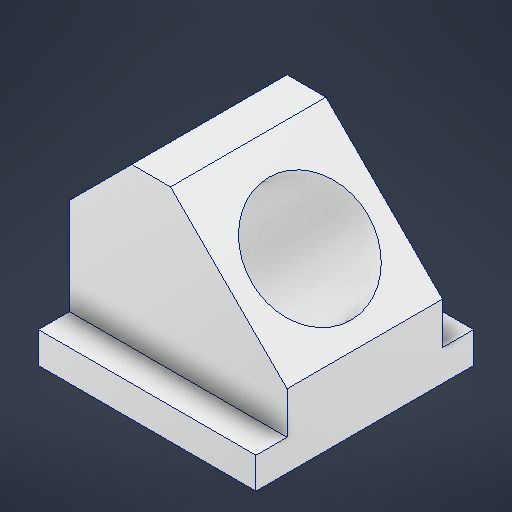
# Autodesk Inventor part: MMAE 232 - Assignment 1a-Nicholas Skiba
Saved by Autodesk Inventor 2026.1 (Build 301233000, 233)
## iProperties
Created: 2025-08-25
Part Number: MMAE 232 - Assignment 1a-Nicholas Skiba
Material: Aluminum 6061
Document SubType Name: Modeling
Designer: Nick
Density: 2.7 g/cm^3
Appearance: Aluminum - Flat
Mass: 20806.1 g
Surface Area: 3990.36 cm^2
Volume: 7705.95 cm^3
Author: Nick
Autodesk Inventor part; units mm, degrees
ref_plane "YZ Plane" through (0, 0, 0) normal (1, 0, 0) x (0, 1, 0)
ref_plane "XZ Plane" through (0, 0, 0) normal (0, 1, 0) x (-1, 0, 0)
ref_plane "XY Plane" through (0, 0, 0) normal (0, 0, 1) x (1, 0, 0)
sketch "Sketch1" plane through (0, 0, 0) normal (0, 1, 0) x (-1, 0, 0)
  line L0 (0, 0) -> (280, 0)
  line L1 (280, 0) -> (280, -280)
  line L2 (280, -280) -> (0, -280)
  line L3 (0, -280) -> (0, 0)
  line L4 (0, 0) -> (0, -20)
  line L5 (0, -20) -> (280, -20)
  line L6 (280, -20) -> (280, -260)
  line L7 (280, -260) -> (0, -260)
  line L8 (0, -260) -> (0, -20)
  dimension "d0" = 280
  dimension "d1" = 280
  dimension "d2" = 20
  dimension "d3" = 240
  constraints: 18 end point, 4 parallel, 2 horizontal, 2 perpendicular, 2 point on line
  measures "d0" distance of L1.end L2.end
  measures "d1" distance of L0.end L1.end
  measures "d2" distance of L0.start L4.end
  measures "d3" distance of L5.end L6.end
extrude "Extrusion1" add sketch "Sketch1" along normal blind 244 contours L5 L1 L7 L3
sketch "Sketch2" plane through (0, 0, 0) normal (0, -1, 0) x (1, 0, 0)
  line L0 (0, 0) -> (-280, 0)
  line L1 (-280, 0) -> (-280, -280)
  line L2 (-280, -280) -> (0, -280)
  line L3 (0, -280) -> (0, 0)
  dimension "d6" = 280
  dimension "d7" = 280
  constraints: 8 end point, 2 parallel, 1 horizontal, 1 perpendicular
  measures "d6" distance of L2.end L1.end
  measures "d7" distance of L1.end L0.end
extrude "Extrusion2" add sketch "Sketch2" against normal blind 40
sketch "Sketch3" plane through (-280, 244, -20) normal (0, 0, 1) x (1, 0, 0)
  line L0 (0, -244) -> (280, -244) projected
  line L1 (0, -244) -> (0, -80)
  line L2 (0, -204) -> (0, 0) projected
  line L3 (0, 0) -> (80, 0)
  line L4 (0, 0) -> (280, 0) projected
  line L5 (80, 0) -> (130, 0)
  line L6 (280, -244) -> (280, -150)
  line L7 (280, -244) -> (280, -204) projected
  line L8 (280, -150) -> (130, 0)
  line L9 (0, -80) -> (80, 0)
  line L10 (0, 0) -> (0, -80)
  line L11 (280, 0) -> (280, -150)
  line L12 (280, 0) -> (130, 0)
  dimension "d10" = 164
  dimension "d11" = 80
  dimension "d12" = 50
  dimension "d13" = 94
  constraints: 18 end point, 4 point on line, 2 collinear, 2 parallel, 1 perpendicular
  measures "d10" distance of L0.start L1.end
  measures "d11" distance of L2.end L3.end
  measures "d12" distance of L3.end L5.end
  measures "d13" distance of L0.end L6.end
extrude "Extrusion3" cut sketch "Sketch3" against normal through all contours L2 L3 L9 | L8 L4 L11
sketch "Sketch4" plane through (-150, 244, -260) normal (0.7071, 0.7071, 0) x (-0.7071, 0.7071, 0)
  line L0 (-212.132, 0) -> (-212.132, 240) projected
  line L1 (-212.132, 240) -> (0, 240) projected
  point P0 (-278.6001, 260)
  point P1 (-112.132, 120)
  dimension "d16" = 100
  dimension "d17" = 120
  measures "d16" distance from line of L0 point (-112.132, 120)
  measures "d17" distance from line of L1 point (-112.132, 120)
hole "Hole1" at (-70.7107, 164.7107, -140) direction (-0.7071, -0.7071, 0) diameter 150 end through all
sketch "Sketch5" plane through (-280, 40, -20) normal (0, 0, 1) x (1, 0, 0)
  line L0 (280, 0) -> (0, 0) projected
  line L1 (0, 0) -> (280, 0)
  line L2 (130, 204) -> (280, 54) projected
  line L3 (280, 0) -> (280, 54)
  line L4 (280, 54) -> (130, 204)
  line L5 (130, 204) -> (80, 204) projected
  line L6 (130, 204) -> (80, 204)
  line L7 (0, 0) -> (0, 124) projected
  line L8 (80, 204) -> (0, 124)
  line L9 (0, 124) -> (0, 0)
  point P0 (280, -40)
  constraints: 12 end point, 3 collinear, 2 perpendicular, 1 horizontal
extrude "Extrusion4" cut sketch "Sketch5" against normal blind 20
sketch "Sketch6" plane through (0, 40, -260) normal (0, 0, -1) x (-1, 0, 0)
  line L0 (0, 0) -> (280, 0) projected
  line L1 (150, 204) -> (0, 54) projected
  line L2 (0, 0) -> (0, 54)
  line L3 (0, 54) -> (150, 204)
  line L4 (280, 124) -> (200, 204) projected
  line L5 (150, 204) -> (200, 204)
  line L6 (200, 204) -> (280, 124)
  line L7 (280, 124) -> (280, 0)
  line L8 (280, 0) -> (0, 0)
  point P0 (0, -40)
  constraints: 12 end point, 2 collinear, 2 perpendicular, 1 parallel, 1 vertical
extrude "Extrusion5" cut sketch "Sketch6" against normal blind 20
body "Solid1"
